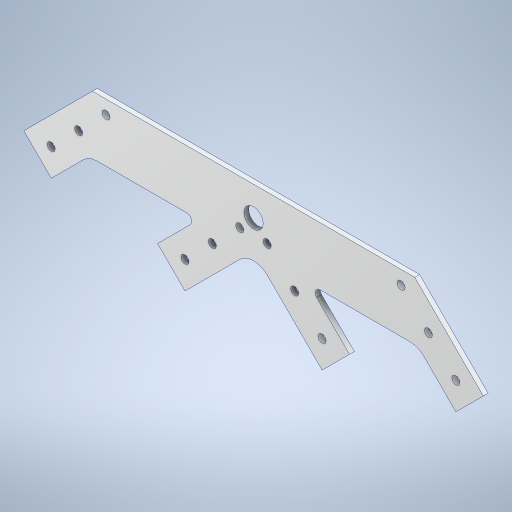
# Autodesk Inventor part: CH1-01-KneePivotPlate
Saved by Autodesk Inventor 2023 (Build 270158000, 158)
## iProperties
Created: 2023-03-03
Part Number: CH1-01-KneePivotPlate
Material: Aluminum 6061
Document SubType Name: Modeling
Designer: megan
Density: 2.7 g/cm^3
Appearance: Aluminum - Flat
Mass: 134.421 g
Surface Area: 352.442 cm^2
Volume: 49.7856 cm^3
Author: megan
Autodesk Inventor part; units mm, degrees
ref_plane "YZ Plane" through (0, 0, 0) normal (1, 0, 0) x (0, 1, 0)
ref_plane "XZ Plane" through (0, 0, 0) normal (0, 1, 0) x (-1, 0, 0)
ref_plane "XY Plane" through (0, 0, 0) normal (0, 0, 1) x (1, 0, 0)
sketch "Sketch1" plane through (0, 0, 0) normal (0, 0, 1) x (1, 0, 0)
  circle A0 centre (0, 0) radius 6.35
  line L0 (-62.8618, -45.9908) -> (-35.921, -19.05)
  line L1 (0, -80.5515) -> (0, 35.6503) projected
  line L2 (0, -19.05) -> (-44.9013, -63.9513)
  line L3 (-44.9013, -63.9513) -> (-62.8618, -45.9908)
  line L4 (0, 19.05) -> (-105.5841, 19.05)
  line L5 (-105.5841, 19.05) -> (-150.4854, -25.8513)
  line L6 (-150.4854, -25.8513) -> (-132.5249, -43.8118)
  line L7 (-132.5249, -43.8118) -> (-107.7631, -19.05)
  line L8 (-107.7631, -19.05) -> (-35.921, -19.05)
  line L9 (62.8618, -45.9908) -> (35.921, -19.05)
  line L10 (0, -19.05) -> (44.9013, -63.9513)
  line L11 (44.9013, -63.9513) -> (62.8618, -45.9908)
  line L12 (0, 19.05) -> (105.5841, 19.05)
  line L13 (105.5841, 19.05) -> (150.4854, -25.8513)
  line L14 (150.4854, -25.8513) -> (132.5249, -43.8118)
  line L15 (132.5249, -43.8118) -> (107.7631, -19.05)
  line L16 (107.7631, -19.05) -> (35.921, -19.05)
  line L17 (0, -19.05) -> (-10.6721, -29.7221)
  point P0 (-62.4057, -45.5347)
  dimension "d1" = 12.7
  dimension "d4" = 63.5
  dimension "d6" = 45
  dimension "d15" = 25.4
  dimension "d59" = 25.4
  dimension "d61" = 101.6
  dimension "d62" = 38.1
  dimension "d63" = 19.05
  dimension "d83" = 19.05
  constraints: 34 end point, 7 symmetric about line, 4 parallel, 4 point on line, 3 perpendicular, 1 centre point, 1 horizontal
  measures "d1" diameter of A0
  measures "d4" distance of L2.start L2.end
  measures "d6" angle of L2 L1
  measures "d15" distance between parallel lines of L2 L0
  measures "d59" distance of L5.end L6.end
  measures "d61" distance between parallel lines of L2 L5
  measures "d62" distance between parallel lines of L8 L4
  measures "d63" distance of point (0, 0) L2.start
  measures "d83" distance from line of L16 point (0, 0)
extrude "Extrusion1" add sketch "Sketch1" along normal blind 3.175 contours A0 L1 L12 L13 L14 L15 L16 L9 L11 L10 | A0 L1 L2 L3 L0 L8 L7 L6 L5 L4
sketch "Sketch3" plane through (0, 0, 3.175) normal (0, 0, 1) x (1, 0, 0)
  line L0 (44.9013, -63.9513) -> (62.8618, -45.9908) projected
  line L1 (62.8618, -45.9908) -> (35.921, -19.05) projected
  line L2 (35.921, -19.05) -> (107.7631, -19.05) projected
  line L3 (107.7631, -19.05) -> (132.5249, -43.8118) projected
  line L4 (132.5249, -43.8118) -> (150.4854, -25.8513) projected
  line L5 (150.4854, -25.8513) -> (105.5841, 19.05) projected
  line L6 (105.5841, 19.05) -> (-105.5841, 19.05) projected
  line L7 (-105.5841, 19.05) -> (-150.4854, -25.8513) projected
  line L8 (-150.4854, -25.8513) -> (-132.5249, -43.8118) projected
  line L9 (-132.5249, -43.8118) -> (-107.7631, -19.05) projected
  line L10 (-107.7631, -19.05) -> (-35.921, -19.05) projected
  line L11 (-35.921, -19.05) -> (-62.8618, -45.9908) projected
  line L12 (-62.8618, -45.9908) -> (-44.9013, -63.9513) projected
  line L13 (-44.9013, -63.9513) -> (0, -19.05) projected
  line L14 (0, -19.05) -> (44.9013, -63.9513) projected
  circle A0 centre (0, 0) radius 6.35 projected
  line L15 (-141.5051, -34.8315) -> (-87.6236, 19.05)
  line L16 (-53.8815, -54.971) -> (20.1395, 19.05)
  circle A1 centre (-132.5249, -25.8513) radius 2.65
  circle A2 centre (-114.5644, -7.8908) radius 2.65
  circle A3 centre (-96.6038, 10.0697) radius 2.65
  circle A4 centre (-44.9013, -45.9908) radius 2.65
  circle A5 centre (-26.9408, -28.0303) radius 2.65
  circle A6 centre (-8.9803, -10.0697) radius 2.65
  dimension "d64" = 5.3
  dimension "d67" = 25.4
  dimension "d72" = 12.7
  dimension "d73" = 12.7
  dimension "d76" = 25.4
  constraints: 6 centre point, 4 end point, 4 point on line, 2 midpoint, 2 parallel, 1 equal radius, 10 other
  measures "d64" diameter of A1
  measures "d67" distance of A1.centre A2.centre
  measures "d72" distance from line of L8 A1.centre
  measures "d73" distance from line of L12 A4.centre
  measures "d76" distance of A4.centre A5.centre
extrude "Extrusion3" cut sketch "Sketch3" against normal blind 25.4 contours A4 L16 | L16 A4 | A5 L16 | L16 A5 | A6 L16 | L16 A6 | A3 L15 | L15 A3 | A1 L15 | L15 A1 | A2 L15 | L15 A2
mirror "Mirror2" about plane through (0, 0, 0) normal (1, 0, 0) of "Extrusion3"
fillet "Fillet1" radius 12.7 3 edges at (-107.7631, -19.05, 1.5875) (0, -19.05, 1.5875) (107.7631, -19.05, 1.5875)
fillet "Fillet2" radius 3.175 2 edges at (-35.921, -19.05, 1.5875) (35.921, -19.05, 1.5875)
sketch "Sketch4" plane through (0, 0, 3.175) normal (0, 0, 1) x (1, 0, 0)
  circle A0 centre (96.6038, 10.0697) radius 2.65 projected
  circle A1 centre (44.9013, -45.9908) radius 2.65 projected
  circle A2 centre (114.5644, -7.8908) radius 2.65 projected
  circle A3 centre (26.9408, -28.0303) radius 2.65 projected
  circle A4 centre (8.9803, -10.0697) radius 2.65 projected
  circle A5 centre (132.5249, -25.8513) radius 2.65 projected
  circle A6 centre (-96.6038, 10.0697) radius 2.65 projected
  circle A7 centre (-44.9013, -45.9908) radius 2.65 projected
  circle A8 centre (-114.5644, -7.8908) radius 2.65 projected
  circle A9 centre (-26.9408, -28.0303) radius 2.65 projected
  circle A10 centre (-8.9803, -10.0697) radius 2.65 projected
  circle A11 centre (-132.5249, -25.8513) radius 2.65 projected
  line L0 (44.9013, -63.9513) -> (62.8618, -45.9908) projected
  line L1 (62.8618, -45.9908) -> (41.3411, -24.4701) projected
  arc A12 (43.5862, -19.05) -> (41.3411, -24.4701) centre (43.5862, -22.225) ccw projected
  line L2 (43.5862, -19.05) -> (102.5026, -19.05) projected
  arc A13 (111.4828, -22.7697) -> (102.5026, -19.05) centre (102.5026, -31.75) ccw projected
  line L3 (111.4828, -22.7697) -> (132.5249, -43.8118) projected
  line L4 (132.5249, -43.8118) -> (150.4854, -25.8513) projected
  line L5 (150.4854, -25.8513) -> (105.5841, 19.05) projected
  line L6 (105.5841, 19.05) -> (-105.5841, 19.05) projected
  line L7 (-105.5841, 19.05) -> (-150.4854, -25.8513) projected
  line L8 (-150.4854, -25.8513) -> (-132.5249, -43.8118) projected
  line L9 (-132.5249, -43.8118) -> (-111.4828, -22.7697) projected
  arc A14 (-102.5026, -19.05) -> (-111.4828, -22.7697) centre (-102.5026, -31.75) ccw projected
  line L10 (-102.5026, -19.05) -> (-43.5862, -19.05) projected
  arc A15 (-41.3411, -24.4701) -> (-43.5862, -19.05) centre (-43.5862, -22.225) ccw projected
  line L11 (-41.3411, -24.4701) -> (-62.8618, -45.9908) projected
  line L12 (-62.8618, -45.9908) -> (-44.9013, -63.9513) projected
  line L13 (-44.9013, -63.9513) -> (-8.9803, -28.0303) projected
  arc A16 (8.9803, -28.0303) -> (-8.9803, -28.0303) centre (0, -37.0105) ccw projected
  line L14 (8.9803, -28.0303) -> (44.9013, -63.9513) projected
  circle A17 centre (0, 0) radius 6.35 projected
  line L15 (-107.7517, -54.9597) -> (0, 52.792)
  line L16 (0, -89.1777) -> (0, 87.4073) projected
  line L17 (0, 52.792) -> (-89.8026, 52.792)
  dimension "d86" = 50.8
  dimension "d87" = 116.7433
  constraints: 4 end point, 1 horizontal, 1 parallel, 1 point on line
  measures "d86" distance between parallel lines of L15 L7
  measures "d87" distance from line of L17 L12.end
equation "\"d6\" = 0.5 * theta12"
equation "\"d59\" = d15"
equation "\"d61\" = gearboxLength"
equation "\"d63\" = 0.5 * d62"
equation "\"d83\" = d63"
equation "\"topDiameter\" = 45"
equation "\"bearingDiameter\" = 28.62"
equation "\"plateThickness\" = 6.35"
equation "\"theta12\" = 90deg"
equation "\"gearboxLength\" = 101.6"
equation "\"boltedLength\" = 76.2"
equation "\"topDiameter_1\" = 25"
equation "\"shaftLength_1\" = 76.2"
equation "\"bearingDiameter_1\" = 28.62"
equation "\"plateThickness_1\" = 6.35"
equation "\"theta12_1\" = 100deg"
equation "\"boltDiameter_1\" = 6"
equation "\"gearboxLength_1\" = 101.6"
equation "\"boltedLength_1\" = 76.2"
equation "\"innerBoltSpacing_1\" = 12.7"
equation "\"outerBoltSpacing_1\" = 12.7"
equation "\"shaftLength\" = 76.2"
equation "\"boltDiameter\" = 5.3"
equation "\"outerBoltSpacing\" = 12.7"
equation "\"innerBoltSpacing\" = 12.7"
body "Solid1"
